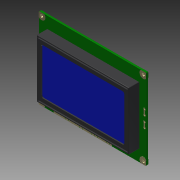
# Autodesk Inventor part: lcd_display
Saved by Autodesk Inventor 2015 (Build 190159000, 159)
## iProperties
Created: 2014-10-13
Part Number: lcd_display
Material: Generic
Document SubType Name: Modeling
Designer: Adam
Density: 1 g/cm^3
Appearance: Gold - Metal
Author: Adam
Autodesk Inventor part; units mm, degrees
ref_plane "YZ Plane" through (0, 0, 0) normal (1, 0, 0) x (0, 1, 0)
sketch "Sketch1" plane through (0, 0, 0) normal (0, 0, 1) x (1, 0, 0)
  line L0 (0, 0) -> (93.05, 0)
  line L1 (93.05, 0) -> (93.05, 70)
  line L2 (93.05, 70) -> (0, 70)
  line L3 (0, 70) -> (0, 0)
  dimension "d0" = 93.05
  dimension "d1" = 70
  constraints: 8 end point, 2 parallel, 1 horizontal, 1 perpendicular
  measures "d0" distance of L0.start L0.end
  measures "d1" distance of L2.end L0.start
extrude "Extrusion1" add sketch "Sketch1" along normal blind 1.6
sketch "Sketch2" plane through (0, 0, 1.6) normal (0, 0, 1) x (1, 0, 0)
  line L0 (7, 60.1) -> (87, 60.1)
  line L1 (87, 60.1) -> (87, 9.9)
  line L2 (87, 9.9) -> (7, 9.9)
  line L3 (7, 9.9) -> (7, 60.1)
  line L4 (93.05, 70) -> (0, 70) projected
  line L5 (0, 70) -> (0, 0) projected
  dimension "d4" = 50.2
  dimension "d5" = 80
  dimension "d6" = 9.9
  dimension "d7" = 7
  constraints: 8 end point, 2 parallel, 1 horizontal, 1 perpendicular
  measures "d4" distance of L2.end L0.start
  measures "d5" distance of L0.start L0.end
  measures "d6" distance between parallel lines of L4 L0
  measures "d7" distance between parallel lines of L5 L3
extrude "Extrusion2" add sketch "Sketch2" along normal blind 9
sketch "Sketch3" plane through (0, 0, 10.6) normal (0, 0, 1) x (1, 0, 0)
  line L0 (11, 55) -> (83, 55)
  line L1 (83, 55) -> (83, 15)
  line L2 (83, 15) -> (11, 15)
  line L3 (11, 15) -> (11, 55)
  line L4 (7, 60.1) -> (7, 9.9) construction
  line L5 (7, 35) -> (87, 35) construction
  line L6 (87, 60.1) -> (87, 9.9) construction
  line L7 (87, 60.1) -> (7, 60.1) construction
  line L8 (47, 60.1) -> (47, 9.9) construction
  line L9 (87, 9.9) -> (7, 9.9) construction
  point P0 (0, 0)
  dimension "d10" = 40
  dimension "d11" = 72
  dimension "d12" = 40
  dimension "d13" = 72
  constraints: 12 end point, 4 midpoint, 2 parallel, 1 horizontal, 1 perpendicular
  measures "d10" distance of L2.end L0.start
  measures "d11" distance of L0.start L0.end
  measures "d12" diameter of L0 L5
  measures "d13" diameter of L3 L8
extrude "Extrusion3" cut sketch "Sketch3" against normal blind 1
fillet "Fillet1" radius 1.5 4 edges at (11, 15, 10.1) (11, 55, 10.1) (83, 55, 10.1) (83, 15, 10.1)
sketch "Sketch4" plane through (0, 0, 10.6) normal (0, 0, 1) x (1, 0, 0)
  line L0 (8, 59.1) -> (86, 59.1)
  line L1 (86, 59.1) -> (86, 58.1)
  line L2 (86, 58.1) -> (8, 58.1)
  line L3 (8, 58.1) -> (8, 59.1)
  line L4 (8, 11.9) -> (86, 11.9)
  line L5 (86, 11.9) -> (86, 10.9)
  line L6 (86, 10.9) -> (8, 10.9)
  line L7 (8, 10.9) -> (8, 11.9)
  line L8 (87, 60.1) -> (7, 60.1) projected
  line L9 (7, 9.9) -> (87, 9.9) projected
  line L10 (7, 9.9) -> (7, 60.1) projected
  line L11 (87, 9.9) -> (87, 60.1) projected
  point P0 (0, 0)
  dimension "d17" = 1
  dimension "d18" = 1
  dimension "d19" = 1
  dimension "d20" = 1
  dimension "d21" = 1
  constraints: 16 end point, 4 parallel, 2 horizontal, 2 perpendicular, 2 point on line, 1 collinear
  measures "d17" distance between parallel lines of L6 L4
  measures "d18" distance between parallel lines of L8 L0
  measures "d19" distance between parallel lines of L9 L6
  measures "d20" distance between parallel lines of L10 L7
  measures "d21" distance between parallel lines of L11 L5
extrude "Extrusion4" cut sketch "Sketch4" against normal up to surface (1 mm away) contours L0 L1 L2 L3 | L4 L5 L6 L7
fillet "Fillet2" radius 0.5 8 edges at (8, 10.9, 10.1) (8, 11.9, 10.1) (86, 10.9, 10.1) (86, 11.9, 10.1) (86, 58.1, 10.1) (86, 59.1, 10.1) (8, 58.1, 10.1) (8, 59.1, 10.1)
fillet "Fillet3" radius 0.5 4 edges at (7, 9.9, 6.1) (7, 60.1, 6.1) (87, 60.1, 6.1) (87, 9.9, 6.1)
sketch "Sketch5" plane through (0, 0, 1.6) normal (0, 0, 1) x (1, 0, 0)
  line L0 (0, 2.5) -> (93.4314, 2.5) construction
  line L1 (2.5, 0) -> (2.5, 70.1679) construction
  line L2 (0, 70) -> (0, 0) construction
  line L3 (0, 67.5) -> (93.0719, 67.5) construction
  line L4 (90.5, 70.1679) -> (90.5, 0) construction
  line L5 (93.05, 70) -> (0, 70) construction
  point P0 (2.5, 67.5)
  point P1 (90.5, 67.5)
  point P2 (90.5, 2.5)
  point P3 (2.5, 2.5)
  dimension "d26" = 2.5
  dimension "d27" = 88
  dimension "d28" = 2.5
  dimension "d29" = 65
  constraints: 10 point on line, 8 end point, 2 horizontal, 2 vertical
  measures "d26" distance between parallel lines of L2 L1
  measures "d27" distance of point (90.5, 2.5) point (2.5, 2.5)
  measures "d28" distance from line of L5 point (90.5, 67.5)
  measures "d29" distance between parallel lines of L0 L3
hole "Hole1" at (2.5, 67.5, 1.6) at (90.5, 67.5, 1.6) at (90.5, 2.5, 1.6) at (2.5, 2.5, 1.6) direction (0, 0, -1) diameter 2.5 end through all
sketch "Sketch6" plane through (0, 0, 1.6) normal (0, 0, 1) x (1, 0, 0)
  line L0 (7.2779, 2.5) -> (62.9327, 2.5) construction
  line L1 (0, 70) -> (0, 0) construction
  line L2 (0, 0) -> (93.05, 0) construction
  point P0 (14, 2.5)
  dimension "d37" = 14
  dimension "d38" = 2.5
  constraints: 2 end point, 1 horizontal, 1 point on line
  measures "d37" distance from line of L1 point (14, 2.5)
  measures "d38" distance from line of L2 point (14, 2.5)
hole "Hole2" at (14, 2.5, 1.6) direction (0, 0, -1) diameter 1 end through all
sketch "Sketch7" plane through (0, 0, 1.6) normal (0, 0, 1) x (1, 0, 0)
  circle A0 centre (14, 2.5) radius 1.143
  circle A1 centre (14, 2.5) radius 0.5 projected
  line L0 (12.857, 2.5) -> (12.857, 0)
  line L1 (12.857, 0) -> (15.143, 0)
  line L2 (15.143, 0) -> (15.143, 2.5)
  line L3 (0, 0) -> (93.05, 0) projected
  dimension "d46" = 2.286
  constraints: 6 end point, 2 perpendicular, 2 point on circle, 2 tangent, 1 centre point, 1 collinear, 1 concentric, 1 vertical
  measures "d46" diameter of A0
extrude "Extrusion5" add sketch "Sketch7" along normal blind 0.1
sketch "Sketch8" plane through (0, 0, 0) normal (0, 0, -1) x (-1, 0, 0)
  circle A0 centre (-14, 2.5) radius 0.5 projected
  line L0 (-12.857, 2.5) -> (-12.857, 0) projected
  line L1 (-12.857, 0) -> (-15.143, 0) projected
  line L2 (-15.143, 0) -> (-15.143, 2.5) projected
  arc A1 (-12.857, 2.5) -> (-15.143, 2.5) centre (-14, 2.5) ccw projected
  point P0 (0, 0)
extrude "Extrusion6" add sketch "Sketch8" along normal blind 0.1
pattern_linear "Rectangular Pattern1" count 20 spacing 2.54 along (1, 0, 0) of "Extrusion6", "Hole2", "Extrusion5"
sketch "Sketch9" plane through (0, 0, 1.6) normal (0, 0, 1) x (1, 0, 0)
  circle A0 centre (2.5, 2.5) radius 1.25 projected
  circle A1 centre (2.5, 67.5) radius 1.25 projected
  circle A2 centre (90.5, 67.5) radius 1.25 projected
  circle A3 centre (90.5, 2.5) radius 1.25 projected
  line L0 (0, 70) -> (0, 0) projected
  line L1 (0, 4.5767) -> (0, 0.4233)
  line L2 (0, 0) -> (12.857, 0) projected
  line L3 (0.4233, 0) -> (4.5767, 0)
  arc A4 (4.5767, 0) -> (0, 4.5767) centre (2.5, 2.5) ccw
  arc A5 (0, 0.4233) -> (0.4233, 0) centre (2.5, 2.5) ccw
  line L4 (0, 65.4233) -> (0, 69.5767)
  line L5 (93.05, 70) -> (0, 70) projected
  line L6 (0.4233, 70) -> (4.5767, 70)
  arc A6 (0.4233, 70) -> (0, 69.5767) centre (2.5, 67.5) ccw
  arc A7 (0, 65.4233) -> (4.5767, 70) centre (2.5, 67.5) ccw
  line L7 (88.4233, 70) -> (92.5767, 70)
  line L8 (93.05, 0) -> (93.05, 70) projected
  line L9 (93.05, 69.5149) -> (93.05, 65.4851)
  arc A8 (93.05, 69.5149) -> (92.5767, 70) centre (90.5, 67.5) ccw
  arc A9 (88.4233, 70) -> (93.05, 65.4851) centre (90.5, 67.5) ccw
  line L10 (88.4233, 0) -> (92.5767, 0)
  line L11 (63.403, 0) -> (93.05, 0) projected
  line L12 (93.05, 0.4851) -> (93.05, 4.5149)
  arc A10 (92.5767, 0) -> (93.05, 0.4851) centre (90.5, 2.5) ccw
  arc A11 (93.05, 4.5149) -> (88.4233, 0) centre (90.5, 2.5) ccw
  dimension "d55" = 3.25
  constraints: 16 end point, 16 point on circle, 15 point on line, 8 centre point, 7 equal radius, 4 coincident, 1 collinear
  measures "d55" radius of A7
extrude "Extrusion7" add sketch "Sketch9" along normal up to surface (0.1 mm away) contours A6 L5 A7 L0 | A4 L2 A5 L0 | A8 L8 A9 L5 | A10 L10 A11 L8
sketch "Sketch10" plane through (0, 0, 0) normal (0, 0, -1) x (-1, 0, 0)
  line L0 (-88.4233, 70) -> (-92.5767, 70) projected
  arc A0 (-93.05, 65.4851) -> (-88.4233, 70) centre (-90.5, 67.5) ccw projected
  line L1 (-93.05, 69.5149) -> (-93.05, 65.4851) projected
  arc A1 (-92.5767, 70) -> (-93.05, 69.5149) centre (-90.5, 67.5) ccw projected
  circle A2 centre (-90.5, 67.5) radius 1.25 projected
  line L2 (0, 65.4233) -> (0, 69.5767) projected
  arc A3 (-4.5767, 70) -> (0, 65.4233) centre (-2.5, 67.5) ccw projected
  line L3 (-0.4233, 70) -> (-4.5767, 70) projected
  arc A4 (0, 69.5767) -> (-0.4233, 70) centre (-2.5, 67.5) ccw projected
  circle A5 centre (-2.5, 67.5) radius 1.25 projected
  circle A6 centre (-90.5, 2.5) radius 1.25 projected
  line L4 (-93.05, 4.5149) -> (-93.05, 0.4851) projected
  arc A7 (-88.4233, 0) -> (-93.05, 4.5149) centre (-90.5, 2.5) ccw projected
  line L5 (-92.5767, 0) -> (-88.4233, 0) projected
  arc A8 (-93.05, 0.4851) -> (-92.5767, 0) centre (-90.5, 2.5) ccw projected
  circle A9 centre (-2.5, 2.5) radius 1.25 projected
  arc A10 (0, 4.5767) -> (-4.5767, 0) centre (-2.5, 2.5) ccw projected
  line L6 (0, 0.4233) -> (0, 4.5767) projected
  arc A11 (-0.4233, 0) -> (0, 0.4233) centre (-2.5, 2.5) ccw projected
  line L7 (-4.5767, 0) -> (-0.4233, 0) projected
  point P0 (0, 0)
extrude "Extrusion8" add sketch "Sketch10" along normal up to surface (0.1 mm away)
chamfer "Chamfer1" distance 0.5 angle 45 4 edges at (93.05, 0, 0.8) (93.05, 70, 0.8) (0, 70, 0.8) (0, 0, 0.8)
sketch "Sketch11" plane through (0, 0, 0) normal (0, 0, -1) x (-1, 0, 0)
  arc A0 (-85.5, 59.1) -> (-85.5, 58.1) centre (-85.5, 58.6) ccw construction
  line L0 (-85.5, 58.1) -> (-8.5, 58.1) construction
  arc A1 (-8.5, 58.1) -> (-8.5, 59.1) centre (-8.5, 58.6) ccw construction
  line L1 (-8.5, 59.1) -> (-85.5, 59.1) construction
  line L2 (-85.5, 10.9) -> (-8.5, 10.9) construction
  arc A2 (-8.5, 10.9) -> (-8.5, 11.9) centre (-8.5, 11.4) ccw construction
  line L3 (-8.5, 11.9) -> (-85.5, 11.9) construction
  arc A3 (-85.5, 11.9) -> (-85.5, 10.9) centre (-85.5, 11.4) ccw construction
  line L4 (-11, 16.5) -> (-11, 53.5) construction
  arc A4 (-11, 53.5) -> (-12.5, 55) centre (-12.5, 53.5) ccw construction
  line L5 (-12.5, 55) -> (-81.5, 55) construction
  arc A5 (-81.5, 55) -> (-83, 53.5) centre (-81.5, 53.5) ccw construction
  line L6 (-83, 53.5) -> (-83, 16.5) construction
  arc A6 (-83, 16.5) -> (-81.5, 15) centre (-81.5, 16.5) ccw construction
  line L7 (-81.5, 15) -> (-12.5, 15) construction
  arc A7 (-12.5, 15) -> (-11, 16.5) centre (-12.5, 16.5) ccw construction
  arc A8 (-87, 10.4) -> (-86.5, 9.9) centre (-86.5, 10.4) ccw construction
  line L8 (-87, 10.4) -> (-87, 59.6) construction
  arc A9 (-86.5, 60.1) -> (-87, 59.6) centre (-86.5, 59.6) ccw construction
  line L9 (-86.5, 60.1) -> (-7.5, 60.1) construction
  arc A10 (-7, 59.6) -> (-7.5, 60.1) centre (-7.5, 59.6) ccw construction
  line L10 (-7, 59.6) -> (-7, 10.4) construction
  arc A11 (-7.5, 9.9) -> (-7, 10.4) centre (-7.5, 10.4) ccw construction
  line L11 (-7.5, 9.9) -> (-86.5, 9.9) construction
  line L12 (-83, 9.9) -> (-78, 9.9)
  line L13 (-78, 9.9) -> (-78, 11.4)
  line L14 (-78, 11.4) -> (-83, 11.4)
  line L15 (-83, 11.4) -> (-83, 9.9)
  line L16 (-83, 60.1) -> (-78, 60.1)
  line L17 (-78, 60.1) -> (-78, 58.6)
  line L18 (-78, 58.6) -> (-83, 58.6)
  line L19 (-83, 58.6) -> (-83, 60.1)
  line L20 (-16, 60.1) -> (-11, 60.1)
  line L21 (-11, 60.1) -> (-11, 58.6)
  line L22 (-11, 58.6) -> (-16, 58.6)
  line L23 (-16, 58.6) -> (-16, 60.1)
  line L24 (-16, 9.9) -> (-11, 9.9)
  line L25 (-11, 9.9) -> (-11, 11.4)
  line L26 (-11, 11.4) -> (-16, 11.4)
  line L27 (-16, 11.4) -> (-16, 9.9)
  point P0 (0, 0)
  dimension "d63" = 1.5
  dimension "d64" = 5
  dimension "d65" = 1.5
  dimension "d67" = 5
  constraints: 32 end point, 8 collinear, 8 parallel, 4 horizontal, 4 perpendicular, 4 point on line
  measures "d63" distance of L14.end L12.start
  measures "d64" distance of L12.start L12.end
  measures "d65" distance between parallel lines of L9 L18
  measures "d67" distance of L24.start L24.end
ref_plane "Work Plane1" through (0, 0, -3) normal (0, 0, 1) x (1, 0, 0)
extrude "Extrusion9" add sketch "Sketch11" along normal up to surface (3 mm away)
sketch "Sketch12" plane through (0, 0, 0) normal (0, 0, -1) x (-1, 0, 0)
  line L0 (-93.05, 4.5149) -> (-93.05, 65.4851) construction
  line L1 (-93.05, 35) -> (0, 35) construction
  line L2 (0, 65.4233) -> (0, 4.5767) construction
  line L3 (-88.4233, 70) -> (-4.5767, 70) construction
  line L4 (-46.5, 70) -> (-46.525, 35) construction
  circle A0 centre (-66.525, 35) radius 7.5
  circle A1 centre (-26.525, 35) radius 7.5
  point P0 (0, 0)
  dimension "d71" = 15
  dimension "d72" = 20
  dimension "d73" = 20
  constraints: 4 end point, 4 midpoint, 2 centre point, 2 point on line, 1 equal radius
  measures "d71" diameter of A0
  measures "d72" distance from line of L4 A1.centre
  measures "d73" distance from line of A0.centre L4
extrude "Extrusion10" add sketch "Sketch12" along normal blind 2
fillet "Fillet4" radius 7.5 2 edges at (74.025, 35, -2) (34.025, 35, -2)
sketch "Sketch13" plane through (0, 0, 9.6) normal (0, 0, 1) x (1, 0, 0)
  arc A0 (81.5, 15) -> (83, 16.5) centre (81.5, 16.5) ccw construction
  line L0 (83, 53.5) -> (83, 16.5) construction
  arc A1 (83, 53.5) -> (81.5, 55) centre (81.5, 53.5) ccw construction
  line L1 (12.5, 55) -> (81.5, 55) construction
  arc A2 (12.5, 55) -> (11, 53.5) centre (12.5, 53.5) ccw construction
  line L2 (11, 16.5) -> (11, 53.5) construction
  arc A3 (11, 16.5) -> (12.5, 15) centre (12.5, 16.5) ccw construction
  line L3 (81.5, 15) -> (12.5, 15) construction
  line L4 (11, 35) -> (83, 35) construction
  line L5 (12.5, 55) -> (81.5, 55) construction
  line L6 (47, 55) -> (47, 15) construction
  line L7 (13.74, 51.62) -> (80.26, 51.62) construction
  line L8 (80.26, 51.62) -> (80.26, 18.38) construction
  line L9 (80.26, 18.38) -> (13.74, 18.38) construction
  line L10 (13.74, 18.38) -> (13.74, 51.62) construction
  line L11 (13.74, 51.62) -> (14.22, 51.62)
  line L12 (14.22, 51.62) -> (14.22, 51.14)
  line L13 (14.22, 51.14) -> (13.74, 51.14)
  line L14 (13.74, 51.14) -> (13.74, 51.62)
  point P0 (0, 0)
  dimension "d77" = 33.24
  dimension "d78" = 66.52
  dimension "d79" = 66.52
  dimension "d80" = 33.24
  dimension "d81" = 0.48
  dimension "d82" = 0.48
  constraints: 20 end point, 4 midpoint, 4 parallel, 2 horizontal, 2 perpendicular
  measures "d77" distance of L9.end L7.start
  measures "d78" distance of L7.start L7.end
  measures "d79" diameter of L10 L6
  measures "d80" diameter of L9 L4
  measures "d81" distance of L7.start L11.end
  measures "d82" distance of L11.end L12.end
extrude "Extrusion11" [suppressed]
fillet "Fillet5" radius 0.5 8 edges at (86.8536, 10.0464, 10.6) (87, 35, 10.6) (86.8536, 59.9536, 10.6) (47, 60.1, 10.6) (7.1464, 59.9536, 10.6) (7, 35, 10.6) (7.1464, 10.0464, 10.6) (47, 9.9, 10.6)
ref_plane "Work Plane2" through (46.525, 4.5767, 1.6) normal (-1, 0, 0) x (0, 0, 1)
sketch "Sketch14" plane through (0, 0, 1.6) normal (0, 0, 1) x (1, 0, 0)
  arc A0 (93.05, 4.5149) -> (88.4233, 0) centre (90.5, 2.5) ccw construction
  line L0 (93.05, 4.5149) -> (93.05, 65.4851) construction
  arc A1 (88.4233, 70) -> (93.05, 65.4851) centre (90.5, 67.5) ccw construction
  line L1 (88.4233, 70) -> (4.5767, 70) construction
  arc A2 (0, 65.4233) -> (4.5767, 70) centre (2.5, 67.5) ccw construction
  line L2 (0, 65.4233) -> (0, 4.5767) construction
  arc A3 (4.5767, 0) -> (0, 4.5767) centre (2.5, 2.5) ccw construction
  line L3 (4.5767, 0) -> (12.857, 0) construction
  line L4 (12.857, 0) -> (12.857, 2.5) construction
  arc A4 (15.143, 2.5) -> (12.857, 2.5) centre (14, 2.5) ccw construction
  line L5 (15.143, 2.5) -> (15.143, 0) construction
  line L6 (15.143, 0) -> (15.397, 0) construction
  line L7 (15.397, 0) -> (15.397, 2.5) construction
  arc A5 (17.683, 2.5) -> (15.397, 2.5) centre (16.54, 2.5) ccw construction
  line L8 (17.683, 2.5) -> (17.683, 0) construction
  line L9 (17.683, 0) -> (17.937, 0) construction
  line L10 (17.937, 0) -> (17.937, 2.5) construction
  arc A6 (20.223, 2.5) -> (17.937, 2.5) centre (19.08, 2.5) ccw construction
  line L11 (20.223, 2.5) -> (20.223, 0) construction
  line L12 (20.223, 0) -> (20.477, 0) construction
  line L13 (20.477, 0) -> (20.477, 2.5) construction
  arc A7 (22.763, 2.5) -> (20.477, 2.5) centre (21.62, 2.5) ccw construction
  line L14 (22.763, 2.5) -> (22.763, 0) construction
  line L15 (22.763, 0) -> (23.017, 0) construction
  line L16 (23.017, 0) -> (23.017, 2.5) construction
  arc A8 (25.303, 2.5) -> (23.017, 2.5) centre (24.16, 2.5) ccw construction
  line L17 (25.303, 2.5) -> (25.303, 0) construction
  line L18 (25.303, 0) -> (25.557, 0) construction
  line L19 (25.557, 0) -> (25.557, 2.5) construction
  arc A9 (27.843, 2.5) -> (25.557, 2.5) centre (26.7, 2.5) ccw construction
  line L20 (27.843, 2.5) -> (27.843, 0) construction
  line L21 (27.843, 0) -> (28.097, 0) construction
  line L22 (28.097, 0) -> (28.097, 2.5) construction
  arc A10 (30.383, 2.5) -> (28.097, 2.5) centre (29.24, 2.5) ccw construction
  line L23 (30.383, 2.5) -> (30.383, 0) construction
  line L24 (30.383, 0) -> (30.637, 0) construction
  line L25 (30.637, 0) -> (30.637, 2.5) construction
  arc A11 (32.923, 2.5) -> (30.637, 2.5) centre (31.78, 2.5) ccw construction
  line L26 (32.923, 2.5) -> (32.923, 0) construction
  line L27 (32.923, 0) -> (33.177, 0) construction
  line L28 (33.177, 0) -> (33.177, 2.5) construction
  arc A12 (35.463, 2.5) -> (33.177, 2.5) centre (34.32, 2.5) ccw construction
  line L29 (35.463, 2.5) -> (35.463, 0) construction
  line L30 (35.463, 0) -> (35.717, 0) construction
  line L31 (35.717, 0) -> (35.717, 2.5) construction
  arc A13 (38.003, 2.5) -> (35.717, 2.5) centre (36.86, 2.5) ccw construction
  line L32 (38.003, 2.5) -> (38.003, 0) construction
  line L33 (38.003, 0) -> (38.257, 0) construction
  line L34 (38.257, 0) -> (38.257, 2.5) construction
  arc A14 (40.543, 2.5) -> (38.257, 2.5) centre (39.4, 2.5) ccw construction
  line L35 (40.543, 2.5) -> (40.543, 0) construction
  line L36 (40.543, 0) -> (40.797, 0) construction
  line L37 (40.797, 0) -> (40.797, 2.5) construction
  arc A15 (43.083, 2.5) -> (40.797, 2.5) centre (41.94, 2.5) ccw construction
  line L38 (43.083, 2.5) -> (43.083, 0) construction
  line L39 (43.083, 0) -> (43.337, 0) construction
  line L40 (43.337, 0) -> (43.337, 2.5) construction
  arc A16 (45.623, 2.5) -> (43.337, 2.5) centre (44.48, 2.5) ccw construction
  line L41 (45.623, 2.5) -> (45.623, 0) construction
  line L42 (45.623, 0) -> (45.877, 0) construction
  line L43 (45.877, 0) -> (45.877, 2.5) construction
  arc A17 (48.163, 2.5) -> (45.877, 2.5) centre (47.02, 2.5) ccw construction
  line L44 (48.163, 2.5) -> (48.163, 0) construction
  line L45 (48.163, 0) -> (48.417, 0) construction
  line L46 (48.417, 0) -> (48.417, 2.5) construction
  arc A18 (50.703, 2.5) -> (48.417, 2.5) centre (49.56, 2.5) ccw construction
  line L47 (50.703, 2.5) -> (50.703, 0) construction
  line L48 (50.703, 0) -> (50.957, 0) construction
  line L49 (50.957, 0) -> (50.957, 2.5) construction
  arc A19 (53.243, 2.5) -> (50.957, 2.5) centre (52.1, 2.5) ccw construction
  line L50 (53.243, 2.5) -> (53.243, 0) construction
  line L51 (53.243, 0) -> (53.497, 0) construction
  line L52 (53.497, 0) -> (53.497, 2.5) construction
  arc A20 (55.783, 2.5) -> (53.497, 2.5) centre (54.64, 2.5) ccw construction
  line L53 (55.783, 2.5) -> (55.783, 0) construction
  line L54 (55.783, 0) -> (56.037, 0) construction
  line L55 (56.037, 0) -> (56.037, 2.5) construction
  arc A21 (58.323, 2.5) -> (56.037, 2.5) centre (57.18, 2.5) ccw construction
  line L56 (58.323, 2.5) -> (58.323, 0) construction
  line L57 (58.323, 0) -> (58.577, 0) construction
  line L58 (58.577, 0) -> (58.577, 2.5) construction
  arc A22 (60.863, 2.5) -> (58.577, 2.5) centre (59.72, 2.5) ccw construction
  line L59 (60.863, 2.5) -> (60.863, 0) construction
  line L60 (60.863, 0) -> (61.117, 0) construction
  line L61 (61.117, 0) -> (61.117, 2.5) construction
  arc A23 (63.403, 2.5) -> (61.117, 2.5) centre (62.26, 2.5) ccw construction
  line L62 (63.403, 2.5) -> (63.403, 0) construction
  line L63 (63.403, 0) -> (88.4233, 0) construction
  line L64 (87, 59.6) -> (87, 10.4) construction
  arc A24 (86.5, 9.9) -> (87, 10.4) centre (86.5, 10.4) ccw construction
  line L65 (86.5, 9.9) -> (7.5, 9.9) construction
  arc A25 (7, 10.4) -> (7.5, 9.9) centre (7.5, 10.4) ccw construction
  line L66 (7, 10.4) -> (7, 59.6) construction
  arc A26 (7.5, 60.1) -> (7, 59.6) centre (7.5, 59.6) ccw construction
  line L67 (7.5, 60.1) -> (86.5, 60.1) construction
  arc A27 (87, 59.6) -> (86.5, 60.1) centre (86.5, 59.6) ccw construction
  line L68 (0, 65.4233) -> (0, 4.5767) construction
  line L69 (0, 35) -> (93.05, 35) construction
  line L70 (93.05, 4.5149) -> (93.05, 65.4851) construction
  circle A28 centre (91.55, 28) radius 0.5
  circle A29 centre (91.55, 42) radius 0.5
  line L71 (91.55, 42) -> (91.55, 28) construction
  circle A30 centre (91.55, 37.54) radius 0.5
  circle A31 centre (91.55, 32.46) radius 0.5
  point P0 (0, 0)
  dimension "d86" = 1
  dimension "d87" = 1.5
  dimension "d88" = 5.08
  dimension "d90" = 5.08
  dimension "d91" = 14
  dimension "d92" = 14
  constraints: 4 centre point, 4 end point, 3 equal radius, 2 midpoint, 2 point on line, 1 perpendicular, 1 vertical
  measures "d86" diameter of A28
  measures "d87" distance between parallel lines of L70 L71
  measures "d88" distance of A30.centre A31.centre
  measures "d90" diameter of A31.centre L69
  measures "d91" distance of L71.start L71.end
  measures "d92" diameter of L71.start L69
extrude "Extrusion12" cut sketch "Sketch14" against normal through all
sketch "Sketch15" plane through (0, 0, 1.6) normal (0, 0, 1) x (1, 0, 0)
  circle A0 centre (91.55, 42) radius 0.5 projected
  circle A1 centre (91.55, 37.54) radius 0.5 projected
  circle A2 centre (91.55, 32.46) radius 0.5 projected
  circle A3 centre (91.55, 28) radius 0.5 projected
  circle A4 centre (91.55, 42) radius 1
  circle A5 centre (91.55, 37.54) radius 1
  circle A6 centre (91.55, 32.46) radius 1
  circle A7 centre (91.55, 28) radius 1
  line L0 (91.05, 41.134) -> (92.05, 41.134)
  line L1 (92.05, 41.134) -> (92.05, 38.406)
  line L2 (92.05, 38.406) -> (91.05, 38.406)
  line L3 (91.05, 38.406) -> (91.05, 41.134)
  line L4 (91.05, 31.594) -> (92.05, 31.594)
  line L5 (92.05, 31.594) -> (92.05, 28.866)
  line L6 (92.05, 28.866) -> (91.05, 28.866)
  line L7 (91.05, 28.866) -> (91.05, 31.594)
  line L8 (91.55, 42) -> (91.55, 28) construction
  point P0 (0, 0)
  dimension "d95" = 2
  dimension "d96" = 1
  dimension "d97" = 1
  constraints: 18 end point, 4 coincident, 4 parallel, 2 horizontal, 2 perpendicular, 2 point on line, 1 vertical, 12 other
  measures "d96" distance between parallel lines of L1 L3
  measures "d97" diameter of L7 L8
extrude "Extrusion13" add sketch "Sketch15" along normal up to surface (0.1 mm away)
sketch "Sketch16" plane through (0, 0, 0) normal (0, 0, -1) x (-1, 0, 0)
  arc A0 (-91.05, 31.594) -> (-92.05, 31.594) centre (-91.55, 32.46) ccw projected
  line L0 (-91.05, 28.866) -> (-91.05, 31.594) projected
  arc A1 (-92.05, 28.866) -> (-91.05, 28.866) centre (-91.55, 28) ccw projected
  line L1 (-92.05, 31.594) -> (-92.05, 28.866) projected
  circle A2 centre (-91.55, 32.46) radius 0.5 projected
  circle A3 centre (-91.55, 28) radius 0.5 projected
  arc A4 (-91.05, 41.134) -> (-92.05, 41.134) centre (-91.55, 42) ccw projected
  line L2 (-91.05, 38.406) -> (-91.05, 41.134) projected
  arc A5 (-92.05, 38.406) -> (-91.05, 38.406) centre (-91.55, 37.54) ccw projected
  line L3 (-92.05, 41.134) -> (-92.05, 38.406) projected
  circle A6 centre (-91.55, 42) radius 0.5 projected
  circle A7 centre (-91.55, 37.54) radius 0.5 projected
  point P0 (0, 0)
extrude "Extrusion14" add sketch "Sketch16" along normal up to surface (0.1 mm away)
sketch "Sketch17" plane through (0, 0, 9.6) normal (0, 0, 1) x (1, 0, 0)
  line L0 (81.5, 15) -> (12.5, 15) projected
  line L1 (24.7801, 49) -> (67.6387, 49) construction
  line L2 (67.6387, 49) -> (67.6387, 19) construction
  line L3 (67.6387, 19) -> (24.7801, 19) construction
  line L4 (24.7801, 19) -> (24.7801, 49) construction
  point P0 (0, 0)
  dimension "d124" = 30
  dimension "d132" = 4
  constraints: 2 other
  measures "d124" distance of L1.end L2.end
  measures "d132" distance between parallel lines of L0 L3
decal "Decal1"
equation "\"d12\" = d10"
equation "\"d13\" = d11"
equation "\"d19\" = d18"
equation "\"d67\" = d64"
equation "\"d73\" = d72"
equation "\"d79\" = d78"
equation "\"d80\" = d77"
equation "\"d90\" = d88"
equation "\"d92\" = d91"
equation "\"d97\" = d96"
body "Solid1"
